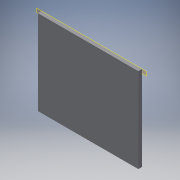
# Autodesk Inventor part: tapa caja
Saved by Autodesk Inventor 2018 (Build 220112000, 112)
## iProperties
Created: 2018-03-07
Part Number: tapa caja
Material: Generic
Document SubType Name: Modeling
Designer: isai
Density: 1 g/cm^3
Appearance: Default
Author: isai
Autodesk Inventor part; units mm, degrees
ref_plane "YZ Plane" through (0, 0, 0) normal (1, 0, 0) x (0, 1, 0)
ref_plane "XZ Plane" through (0, 0, 0) normal (0, 1, 0) x (-1, 0, 0)
ref_plane "XY Plane" through (0, 0, 0) normal (0, 0, 1) x (1, 0, 0)
ref_plane "Work Plane1" through (0, 89, 0) normal (0, 0, 1) x (1, 0, 0)
sketch "Sketch1" plane through (0, 89, 0) normal (0, 0, 1) x (1, 0, 0)
  line L0 (110, -89) -> (0, -89)
  line L1 (0, -89) -> (0, 4)
  line L2 (0, 4) -> (110, 4)
  line L3 (110, 4) -> (110, -89)
  point P0 (0, -89)
  constraints: 8 end point, 2 parallel, 1 horizontal, 1 perpendicular, 2 other
extrude "Extrusion1" add sketch "Sketch1" along normal blind 4
sketch "Sketch2" plane through (0, 89, 4) normal (0, 0, 1) x (1, 0, 0)
  line L0 (0, -89) -> (110, -89) projected
  line L1 (110, -89) -> (110, 4) projected
  line L2 (110, 4) -> (0, 4) projected
  line L3 (0, 4) -> (0, -89) projected
  line L4 (0, -20) -> (0, -10)
  line L5 (4, -10) -> (4, -20)
  line L6 (0, -75) -> (0, -65)
  line L7 (4, -65) -> (4, -75)
  line L8 (0, -65) -> (4, -65)
  line L9 (0, -75) -> (4, -75)
  line L10 (106, -75) -> (106, -65)
  line L11 (110, -65) -> (110, -75)
  line L12 (110, -10) -> (106, -10)
  line L13 (110, -20) -> (106, -20)
  line L14 (106, -20) -> (106, -10)
  line L15 (110, -10) -> (110, -20)
  line L16 (0, 4) -> (110, 4)
  line L17 (110, 4) -> (110, -89)
  line L18 (110, -89) -> (0, -89)
  line L19 (0, -89) -> (0, 4)
  line L20 (0, 4) -> (0, -89) projected
  line L21 (4, -20) -> (0, -20)
  line L22 (0, -20) -> (0, -10)
  line L23 (0, -10) -> (4, -10)
  line L24 (4, -10) -> (4, -20)
  line L25 (0, -75) -> (4, -75)
  line L26 (4, -75) -> (4, -65)
  line L27 (4, -65) -> (0, -65)
  line L28 (0, -65) -> (0, -75)
  line L29 (106, -65) -> (110, -65)
  line L30 (110, -65) -> (110, -75)
  line L31 (110, -75) -> (106, -75)
  line L32 (106, -75) -> (106, -65)
  line L33 (106, -10) -> (110, -10)
  line L34 (110, -10) -> (110, -20)
  line L35 (110, -20) -> (106, -20)
  line L36 (106, -20) -> (106, -10)
  constraints: 64 end point, 10 parallel, 5 horizontal, 5 perpendicular, 1 coincident, 1 other
body "Solid1"
